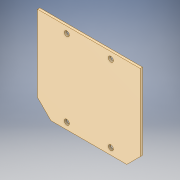
# Autodesk Inventor part: DPLX_P031_VIPE Insulation Top
Saved by Autodesk Inventor 2018 (Build 220112000, 112)
## iProperties
Created: 2017-12-19
Part Number: DPLX_P031_VIPE Insulation Top
Material: Polyethylene, High Density
Document SubType Name: Modeling
Designer: Sam
Density: 0.952 g/cm^3
Appearance: Smooth - Off-White
Mass: 5.71259 g
Surface Area: 83.131 cm^2
Volume: 6.00062 cm^3
Author: Sam
Comments: http://www.eplastics.com/Plastic/G9-G10-FR4-glass-epoxy-sheet/G10NAT-060X12X12
Autodesk Inventor part; units mm, degrees
ref_plane "YZ Plane" through (0, 0, 0) normal (1, 0, 0) x (0, 1, 0)
ref_plane "XZ Plane" through (0, 0, 0) normal (0, 1, 0) x (-1, 0, 0)
ref_plane "XY Plane" through (0, 0, 0) normal (0, 0, 1) x (1, 0, 0)
sketch "Sketch1" plane through (0, 0, 0) normal (0, 0, 1) x (1, 0, 0)
  line L0 (-34.036, -29.7688) -> (34.036, -29.7688)
  line L1 (34.036, -29.7688) -> (34.036, 29.7688)
  line L2 (34.036, 29.7688) -> (-34.036, 29.7688)
  line L3 (-34.036, 29.7688) -> (-34.036, -29.7688)
  line L4 (-34.036, -29.7688) -> (34.036, 29.7688) construction
  line L5 (34.036, -29.7688) -> (-34.036, 29.7688) construction
  point P0 (0, 0)
  dimension "d0" = 68.072
  dimension "d1" = 59.5376
  constraints: 12 end point, 2 midpoint, 2 parallel, 1 horizontal, 1 perpendicular
  measures "d0" distance of L2.end L1.end
  measures "d1" distance of L1.end L0.end
extrude "Extrusion1" add sketch "Sketch1" along normal blind 1.524
chamfer "Chamfer1" distance 8.89 angle 45 2 edges at (-34.036, -29.7688, 0.762) (34.036, -29.7688, 0.762)
sketch "Sketch3" plane through (0, 0, 0) normal (0, 0, -1) x (-1, 0, 0)
  circle A0 centre (-14.605, -25.4024) radius 1.7018 projected
  circle A1 centre (14.605, -25.4024) radius 1.7018 projected
  circle A2 centre (14.605, 25.3976) radius 1.7018 projected
  circle A3 centre (-14.605, 25.3976) radius 1.7018 projected
  point P0 (0, 0)
hole "Hole2" at (14.605, -25.4024, 0) at (-14.605, -25.4024, 0) at (-14.605, 25.3976, 0) at (14.605, 25.3976, 0) direction (0, 0, 1) diameter 3.4036 end through all clearance for "Flat Head Machine Screw" size "M3" standard "Ansi Metric M Profile"
body "Solid1"
